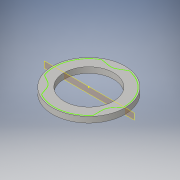
# Autodesk Inventor part: vexCam6
Saved by Autodesk Inventor 2016 SP1 (Build 200210100, 210)
## iProperties
Created: 2015-11-01
Part Number: vexCam6
Material: Generic
Document SubType Name: Modeling
Designer: steele
Density: 1 g/cm^3
Appearance: Default
d6: 20.000 ul
insideDiam: 4.330 in
outsideDiam: 6.330 in
d7: 60.000 ul
d8: 60.000 ul
d9: 140.000 ul
d10: 140.000 ul
d11: 180.000 ul
d12: 180.000 ul
d13: 260.000 ul
d14: 260.000 ul
d15: 300.000 ul
d16: -60.000 ul
d17: 20.000 ul
d5: 0.00 deg
plateThickness: 0.500 in
outerCamRadius: 3.040 in
camMovement: 0.750 in
insideRadius: 2.165 in
ringThickness: 1.000 in
maxCamRunner: 0.250 in
outsideRadius: 3.165 in
Author: steele
Autodesk Inventor part; units mm, degrees
ref_plane "YZ Plane" through (0, 0, 0) normal (1, 0, 0) x (0, 1, 0)
ref_plane "XZ Plane" through (0, 0, 0) normal (0, 1, 0) x (-1, 0, 0)
sketch "Sketch1" plane through (0, 0, 0) normal (0, 1, 0) x (-1, 0, 0)
  point P0 (0, 0)
  point P1 (-59.1499, 49.6362)
  point P2 (72.5603, 26.4121)
  point P3 (38.609, 66.8737)
  point P4 (-77.215, 0.0027)
  point P5 (-13.4074, -76.0402)
  point P6 (-13.4084, -76.0429)
  point P7 (38.608, -66.871)
  point P8 (72.5593, 26.4094)
  constraints: 18 other
sketch "Sketch2" plane through (0, 0, 0) normal (0, 1, 0) x (-1, 0, 0)
  circle A0 centre (0, 0) radius 54.991
  circle A1 centre (0, 0) radius 80.391
  dimension "insideDiam" = 109.982
  dimension "outsideDiam" = 160.782
  constraints: 2 centre point, 2 coincident
  measures "insideDiam" diameter of A0
  measures "outsideDiam" diameter of A1
extrude "Extrusion1" add sketch "Sketch2" against normal blind 12.7
equation "\"outerCamRadius\" = 77.216"
equation "\"outsideRadius\" = 80.391"
equation "\"maxCamRunner\" = 6.35"
equation "\"camMovement\" = 19.05"
equation "\"ringThickness\" = 25.4"
equation "\"insideRadius\" = 54.991"
body "Solid1"
